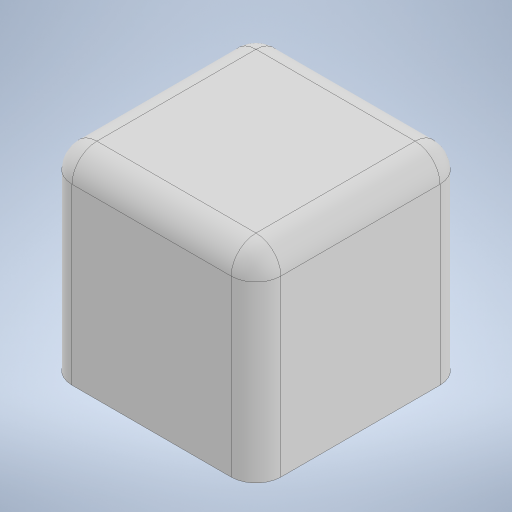
# Autodesk Inventor part: motoreù
Saved by Autodesk Inventor 2024 (Build 280153000, 153)
## iProperties
Created: 2024-03-01
Part Number: motoreù
Material: Generico
Document SubType Name: Modeling
Designer: Giorgio
Density: 1 g/cm^3
Appearance: Default
Author: Giorgio
Autodesk Inventor part; units mm, degrees
ref_plane "YZ Plane" through (0, 0, 0) normal (1, 0, 0) x (0, 1, 0)
ref_plane "XZ Plane" through (0, 0, 0) normal (0, 1, 0) x (-1, 0, 0)
ref_plane "XY Plane" through (0, 0, 0) normal (0, 0, 1) x (1, 0, 0)
sketch "Schizzo1" plane through (0, 0, 0) normal (0, 1, 0) x (-1, 0, 0)
  line L0 (-6.2923, 42) -> (-38.2923, 42)
  line L1 (-43.2923, 37) -> (-43.2923, 5)
  line L2 (-38.2923, 0) -> (-6.2923, 0)
  line L3 (-1.2923, 5) -> (-1.2923, 37)
  arc A0 (-1.2923, 37) -> (-6.2923, 42) centre (-6.2923, 37) ccw
  arc A1 (-38.2923, 42) -> (-43.2923, 37) centre (-38.2923, 37) ccw
  arc A2 (-43.2923, 5) -> (-38.2923, 0) centre (-38.2923, 5) ccw
  arc A3 (-6.2923, 0) -> (-1.2923, 5) centre (-6.2923, 5) ccw
  point P0 (0, 0)
  point P1 (-1.2923, 42)
  point P2 (-43.2923, 0)
  point P3 (-1.2923, 0)
  dimension "d0" = 42
  dimension "d1" = 42
  dimension "d2" = 5
  dimension "d3" = 5
  constraints: 8 end point, 8 point on circle, 8 tangent, 6 point on line, 4 centre point, 2 equal radius, 2 parallel, 1 horizontal, 1 perpendicular
  measures "d0" distance of point (-1.292, 0) point (-1.292, 42)
  measures "d1" distance of point (-43.292, 0) point (-1.292, 0)
  measures "d2" radius of A0
  measures "d3" radius of A1
extrude "Estrusione1" add sketch "Schizzo1" along normal blind 40
fillet "Raccordo1" radius 5 8 edges at (22.2923, 40, 42) (41.8278, 40, 40.5355) (43.2923, 40, 21) (41.8278, 40, 1.4645) (22.2923, 40, 0) (2.7568, 40, 1.4645) (1.2923, 40, 21) (2.7568, 40, 40.5355)
